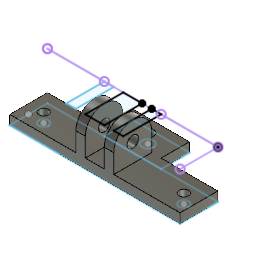
camera_joint_female (Autodesk Fusion 360 design; units mm, degrees)
Autodesk Fusion 360 part; units mm, degrees
note: some values were not read from the file. Set by a fixed rule: which sketch regions a step uses.
sketch "Sketch1" plane through (0, 0, 0) normal (0, 0, 1) x (1, 0, 0)
  line L0 (-20, 30) -> (70, 30)
  line L1 (70, 30) -> (70, 10)
  line L2 (70, 10) -> (-20, 10)
  line L3 (-20, 10) -> (-20, 30)
  circle A0 centre (-12, 20) radius 2.5
  circle A1 centre (62, 20) radius 2.5
  circle A2 centre (25, 37.96) radius 3
  line L4 (40, 30) -> (10, 30)
  line L5 (10, 30) -> (10, 45)
  line L6 (10, 45) -> (40, 45)
  line L7 (40, 45) -> (40, 30)
  point P0 (-20, 20)
  dimension "d31" = 5
  dimension "d32" = 5
  dimension "d33" = 74
  dimension "d37" = 10
  dimension "d38" = 10
  dimension "d47" = 6
  dimension "d48" = 17.96
  constraint horizontal L0
  constraint vertical L1
  constraint horizontal L2
  constraint vertical L3
  constraint horizontal L4
  constraint vertical L5
  constraint horizontal L6
  constraint vertical L7
  constraint coincident L0 L4.start
  measures "d31" diameter of A0
  measures "d32" diameter of A1
  measures "d33" distance of A0.centre A1.centre
  measures "d37" distance of L0 A1.centre
  measures "d38" distance of L2 A1.centre
  measures "d47" diameter of A2
  measures "d48" vertical distance of A1.centre A2.centre
extrude "Extrude1" add sketch "Sketch1" along normal blind 10
sketch "Sketch2" plane through (0, 0, 10) normal (0, 0, 1) x (-1, 0, 0)
  line L0 (20, -10) -> (-70, -10)
  line L1 (-70, -10) -> (-70, -30)
  line L2 (-10, -30) -> (20, -30)
  line L3 (20, -30) -> (20, -10)
  line L4 (-10, -30) -> (-40, -30)
  line L5 (-40, -30) -> (-40, -10)
  line L6 (-40, -10) -> (-10, -10)
  line L7 (-10, -10) -> (-10, -30)
  circle A0 centre (12, -20) radius 2.5
  circle A1 centre (-62, -20) radius 2.5
  circle A2 centre (-25, -37.96) radius 3
  line L8 (-40, -45) -> (-10, -45)
  line L9 (-10, -45) -> (-10, -30)
  line L10 (-70, -30) -> (-40, -30)
  line L11 (-40, -30) -> (-40, -45)
  dimension "d12" = 20
  dimension "d13" = 30
  dimension "d15" = 30
  constraint horizontal L4
  constraint vertical L5
  constraint horizontal L6
  constraint vertical L7
  constraint coincident L2 L4.end
  measures "d12" distance of L2.start L6.end
  measures "d13" distance of L2.start L4.end
  measures "d15" distance of L1 L5
extrude "Extrude2" add sketch "Sketch2" along normal blind 15 contours L0 L4 L5 L6 L7
extrude "Extrude5" add 1 faces at (30, 16.6667, 25) along direction (0, 0, 1) blind 5
sketch "Sketch3" plane through (40, 0, 0) normal (1, 0, 0) x (0, 1, 0)
  line L0 (10, 10) -> (30, 10)
  line L1 (30, 10) -> (30, 30)
  line L2 (10, 30) -> (10, 10)
  circle A0 centre (20, 15) radius 3
  circle A1 centre (20, 15) radius 10
  line L3 (30, 30) -> (10, 30)
  line L4 (10, 10) -> (30, 10)
  dimension "d18" = 6
  dimension "d28" = 5
  constraint concentric A0 A1
  constraint tangent L1 A1
  measures "d18" diameter of A0
  measures "d28" distance of A0.centre L4
extrude "Extrude3" cut sketch "Sketch3" against normal blind 30 contours L1 L2 A1 L3 | A0
ref_plane "WorkPlane1" through (26.6123, 20, 25) normal (0, 0, 1) x (0, -1, 0)
sketch "Sketch4" plane through (0, 0, 25) normal (0, 0, 1) x (1, 0, 0)
  line L0 (20, 30) -> (30, 30)
  line L1 (30, 30) -> (30, 10)
  line L2 (30, 10) -> (20, 10)
  line L3 (20, 10) -> (20, 30)
  line L4 (-20, 30) -> (70, 30)
  line L5 (70, 30) -> (70, 10)
  line L6 (35, 30) -> (40, 30)
  line L7 (40, 30) -> (40, 10)
  line L8 (40, 10) -> (35, 10)
  line L9 (35, 10) -> (35, 30)
  line L10 (10, 30) -> (15, 30)
  line L11 (15, 30) -> (15, 10)
  line L12 (15, 10) -> (10, 10)
  line L13 (10, 10) -> (10, 30)
  line L14 (70, 30) -> (40, 30)
  line L15 (10, 30) -> (-20, 30)
  dimension "d22" = 20
  dimension "d39" = 10
  dimension "d40" = 40
  dimension "d41" = 5
  dimension "d42" = 5
  dimension "d43" = 20
  dimension "d44" = 5
  constraint horizontal L0
  constraint vertical L1
  constraint horizontal L2
  constraint vertical L3
  constraint coincident L0.end L4
  constraint horizontal L6
  constraint vertical L7
  constraint horizontal L8
  constraint vertical L9
  constraint coincident L4 L6.start
  constraint horizontal L10
  constraint vertical L11
  constraint horizontal L12
  constraint vertical L13
  measures "d22" distance of L0.start L2.end
  measures "d39" distance of L0.start L0.end
  measures "d40" distance of L1 L5
  measures "d41" distance of L10.start L10.end
  measures "d42" distance of L7.end L8.end
  measures "d43" distance of L6.end L7.end
  measures "d44" distance of L1 L9
extrude "Extrude4" cut sketch "Sketch4" against normal blind 20 contours L0 L1 L2 L3 L4
extrude "Extrude7" cut sketch "Sketch4" against normal blind 20
extrude "Extrude6" cut 3 faces at (15.6667, 37.6533, 10) (46.5, 20, 10) (3.5, 20, 10) along direction (0, 0, -1) blind 5
fillet "Fillet1" [rolled back] radius 8
